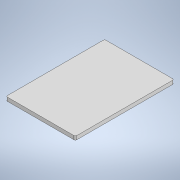
# Autodesk Inventor part: klapka1
Saved by Autodesk Inventor 2021 (Build 250183000, 183)
## iProperties
Created: 2025-11-23
Part Number: klapka1
Material: Ogólny
Document SubType Name: Modeling
Designer: humus
Density: 1 g/cm^3
Appearance: Domyślna
Author: humus
Autodesk Inventor part; units mm, degrees
ref_plane "YZ Plane" through (0, 0, 0) normal (1, 0, 0) x (0, 1, 0)
ref_plane "XZ Plane" through (0, 0, 0) normal (0, 1, 0) x (-1, 0, 0)
ref_plane "XY Plane" through (0, 0, 0) normal (0, 0, 1) x (1, 0, 0)
sketch "Szkic2" plane through (0, 0, 0) normal (0, 1, 0) x (-1, 0, 0)
  line L0 (0, 0) -> (-190, 0)
  line L1 (-190, 0) -> (-190, 270)
  line L2 (-190, 270) -> (0, 270)
  line L3 (0, 270) -> (0, 0)
  dimension "d0" = 190
  dimension "d1" = 270
  constraints: 8 end point, 2 parallel, 1 horizontal, 1 perpendicular
  measures "d0" distance of L1.end L2.end
  measures "d1" distance of L0.end L1.end
extrude "Wyciągnięcie proste1" add sketch "Szkic2" along normal mid plane 10
fillet "Zaokrąglenie1" radius 4 4 edges at (190, 0, 0) (0, 0, 0) (0, 0, 270) (190, 0, 270)
sketch "Szkic4" plane through (0, 0, 0) normal (0, 1, 0) x (-1, 0, 0)
  line L0 (-4, 4) -> (-186, 4)
  line L1 (-186, 4) -> (-186, 266)
  line L2 (-186, 266) -> (-4, 266)
  line L3 (-4, 266) -> (-4, 4)
  line L4 (-186, 0) -> (-4, 0) projected
  line L5 (0, 4) -> (0, 266) projected
  line L6 (-190, 266) -> (-190, 4) projected
  line L7 (-4, 270) -> (-186, 270) projected
  point P0 (0, 0)
  dimension "d13" = 4
  dimension "d14" = 4
  dimension "d16" = 4
  dimension "d17" = 4
  constraints: 8 end point, 2 parallel, 1 horizontal, 1 perpendicular
  measures "d13" distance between parallel lines of L4 L0
  measures "d14" distance between parallel lines of L5 L3
  measures "d16" distance between parallel lines of L6 L1
  measures "d17" distance between parallel lines of L7 L2
extrude "Wyciągnięcie proste3" cut sketch "Szkic4" against normal blind 5
